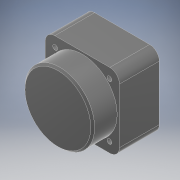
# Autodesk Inventor part: YDLiDAR_T-mini-pro
Saved by Autodesk Inventor 2022.5 (Build 265521000, 521)
## iProperties
Created: 2024-01-14
Part Number: YDLiDAR_T-mini-pro
Material: 一般
Document SubType Name: Modeling
Designer: 8326d
Density: 1 g/cm^3
Appearance: 滑らか - 黒
Author: 8326d
Autodesk Inventor part; units mm, degrees
ref_plane "YZ Plane" through (0, 0, 0) normal (1, 0, 0) x (0, 1, 0)
ref_plane "XZ Plane" through (0, 0, 0) normal (0, 1, 0) x (-1, 0, 0)
ref_plane "XY Plane" through (0, 0, 0) normal (0, 0, 1) x (1, 0, 0)
sketch "スケッチ1" plane through (0, 0, 0) normal (0, 0, 1) x (1, 0, 0)
  line L0 (-19.3, -19.3) -> (19.3, -19.3)
  line L1 (19.3, -19.3) -> (19.3, 19.3)
  line L2 (19.3, 19.3) -> (-19.3, 19.3)
  line L3 (-19.3, 19.3) -> (-19.3, -19.3)
  line L4 (-19.3, -19.3) -> (19.3, 19.3) construction
  line L5 (19.3, -19.3) -> (-19.3, 19.3) construction
  point P0 (0, 0)
  dimension "d0" = 38.6
  dimension "d1" = 38.6
  constraints: 12 end point, 2 midpoint, 2 parallel, 1 horizontal, 1 perpendicular
  measures "d0" distance of L2.end L1.end
  measures "d1" distance of L1.end L0.end
extrude "押し出し1" add sketch "スケッチ1" along normal blind 20.7
sketch "スケッチ2" plane through (0, 0, 20.7) normal (0, 0, 1) x (1, 0, 0)
  circle A0 centre (0, 0) radius 18.1
  dimension "d4" = 36.2
  constraints: 1 centre point, 1 coincident
  measures "d4" diameter of A0
extrude "押し出し2" add sketch "スケッチ2" along normal blind 12.7
sketch "スケッチ3" plane through (0, 0, 0) normal (0, 0, -1) x (-1, 0, 0)
  line L0 (-14.1, -14.1) -> (14.1, -14.1) construction
  line L1 (14.1, -14.1) -> (14.1, 14.1) construction
  line L2 (14.1, 14.1) -> (-14.1, 14.1) construction
  line L3 (-14.1, 14.1) -> (-14.1, -14.1) construction
  line L4 (-14.1, -14.1) -> (14.1, 14.1) construction
  line L5 (14.1, -14.1) -> (-14.1, 14.1) construction
  point P0 (0, 0)
  dimension "d7" = 28.2
  dimension "d8" = 28.2
  constraints: 12 end point, 2 midpoint, 2 parallel, 1 horizontal, 1 perpendicular
  measures "d7" distance of L2.end L1.end
  measures "d8" distance of L1.end L0.end
hole "穴1" at (-14.1, 14.1, 0) at (-14.1, -14.1, 0) at (14.1, -14.1, 0) at (14.1, 14.1, 0) direction (0, 0, 1) diameter 2.5 end through all
fillet "フィレット1" radius 5 4 edges at (19.3, 19.3, 10.35) (19.3, -19.3, 10.35) (-19.3, 19.3, 10.35) (-19.3, -19.3, 10.35)
chamfer "面取り1" distance 1 angle 45 1 edges at (-18.1, 0, 33.4)
